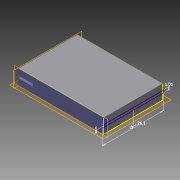
# Autodesk Inventor part: camera_support_on_carbon_blade
Saved by Autodesk Inventor 2015 SP1 (Build 190203100, 203)
## iProperties
Created: 2015-07-01
Part Number: camera_support_on_carbon_blade
Material: Generic
Document SubType Name: Modeling
Designer: Alexandre Cherpillod
Density: 1 g/cm^3
Appearance: Default
Author: Alexandre Cherpillod
Autodesk Inventor part; units mm, degrees
sketch "Sketch1" plane through (0, 0, 0) normal (0, 0, 1) x (1, 0, 0)
  line L0 (0, 0) -> (36, 0)
  line L1 (36, 0) -> (36, 25)
  line L2 (36, 25) -> (0, 25)
  line L3 (0, 25) -> (0, 0)
  dimension "d0" = 36
  dimension "d1" = 25
  constraints: 8 end point, 2 parallel, 1 horizontal, 1 perpendicular
  measures "d0" distance of L2.end L1.end
  measures "d1" distance of L1.end L0.end
extrude "Extrusion1" add sketch "Sketch1" along normal blind 6
sketch "Sketch2" plane through (0, 0, 0) normal (-1, 0, 0) x (0, 0, 1)
  line L0 (0, 0) -> (6, 0) projected
  line L1 (0, 25) -> (6, 25) projected
  line L2 (2.495, 0) -> (3.505, 0)
  line L3 (3.505, 0) -> (3.505, 25)
  line L4 (3.505, 25) -> (2.495, 25)
  line L5 (2.495, 25) -> (2.495, 0)
  point P0 (3, 0)
  point P1 (3, 0)
  dimension "d4" = 0
  dimension "d5" = 1.01
  constraints: 8 end point, 3 midpoint, 2 parallel, 2 point on line, 1 horizontal, 1 perpendicular
  measures "d4" distance of point (3, 0) point (3, 0)
  measures "d5" distance between parallel lines of L3 L5
extrude "Extrusion2" cut sketch "Sketch2" against normal blind 6
sketch "Sketch3" plane through (36, 0, 0) normal (1, 0, 0) x (0, 0, -1)
  line L0 (0, 25) -> (-6, 25) projected
  line L1 (-3.505, -0.55) -> (-2.495, -0.55)
  line L2 (-2.495, -0.55) -> (-2.495, 25.55)
  line L3 (0, 0) -> (-6, 0) projected
  line L4 (0, 0) -> (0, 25) projected
  line L5 (-3.505, -0.55) -> (-3.505, 25.55)
  line L6 (-3.505, 25.55) -> (-2.495, 25.55)
  point P0 (-3.505, 0)
  point P1 (-2.495, 0)
  point P2 (-3, -0.55)
  point P3 (-3, 0)
  point P4 (0, 12.5)
  point P5 (-2.495, 12.5)
  dimension "d11" = 26.1
  dimension "d13" = 0
  dimension "d14" = 0
  dimension "d15" = 1.01
  constraints: 8 end point, 4 midpoint, 2 parallel, 2 perpendicular, 1 horizontal
  measures "d11" distance of L2.end L1.end
  measures "d13" vertical distance of point (0, 12.5) point (-2.495, 12.5)
  measures "d14" horizontal distance of point (-3, 0) point (-3, -0.55)
  measures "d15" distance between parallel lines of L2 L5
body "Solid1"
